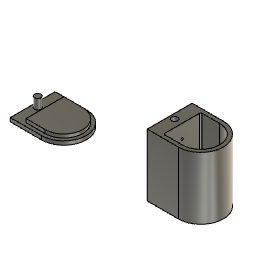
Motor Holder large v1 (Autodesk Fusion 360 design; units mm, degrees)
Autodesk Fusion 360 part; units mm, degrees
sketch "Sketch1" plane through (0, 0, 0) normal (0, 0, 1) x (1, 0, 0)
  line L0 (0, 0) -> (0, 36)
  line L1 (0, 18) -> (18, 18) construction
  circle A0 centre (18, 18) radius 18
  line L2 (0, 36) -> (18, 36)
  line L3 (0, 0) -> (18, 0)
  circle A1 centre (18, 18) radius 1
  circle A2 centre (97.408, 18) radius 1
  line L4 (79.408, 18) -> (97.408, 18) construction
  line L5 (79.408, 36) -> (97.408, 36)
  line L6 (79.408, 0) -> (79.408, 36)
  circle A3 centre (97.408, 18) radius 18
  line L7 (79.408, 0) -> (97.408, 0)
  line L8 (0, 0) -> (-7, 0)
  line L9 (-7, 0) -> (-7, 36)
  line L10 (-7, 36) -> (0, 36)
  line L11 (-117, 0) -> (-117, 36)
  line L12 (-117, 36) -> (-110, 36)
  line L13 (-110, 0) -> (-92, 0)
  line L14 (-110, 0) -> (-117, 0)
  circle A4 centre (-92, 18) radius 18
  line L15 (-110, 18) -> (-92, 18) construction
  line L16 (-110, 0) -> (-110, 36)
  line L17 (-110, 36) -> (-92, 36)
  point P0 (79.408, 0)
  point P1 (-110, 0)
  dimension "d1" = 36
  dimension "d2" = 18
  dimension "d8" = 2
  dimension "d21" = 36
  dimension "d22" = 18
  dimension "d23" = 2
  dimension "d24" = 7
  dimension "d25" = 36
  dimension "d26" = 18
  dimension "d28" = 7
  constraint vertical L0
  constraint coincident L0.start L3.start
  constraint midpoint L0 L1.start
  constraint perpendicular L0 L1
  constraint coincident L1.end A0.centre
  constraint coincident L1.start A0
  constraint coincident A0 L2.end
  constraint tangent A0 L2
  constraint coincident A0 L3.end
  constraint tangent A0 L3
  constraint concentric A0 A1
  constraint vertical L6
  constraint coincident P0 L6.start
  constraint midpoint L4.start L6
  constraint perpendicular L4 L6
  constraint coincident A2.centre L4.end
  constraint coincident L4.start A3
  constraint coincident L5.end A3
  constraint tangent L5 A3
  constraint coincident L7.end A3
  constraint tangent A3 L7
  constraint concentric A2 A3
  constraint perpendicular L0 L8
  constraint perpendicular L8 L9
  constraint vertical L16
  constraint coincident P1 L13.start
  constraint midpoint L15.start L16
  constraint perpendicular L15 L16
  constraint coincident A4.centre L15.end
  constraint coincident L15.start A4
  constraint coincident L17.end A4
  constraint tangent A4 L17
  constraint coincident L13.end A4
  constraint tangent L13 A4
  constraint perpendicular L14 L16
  constraint perpendicular L11 L14
  measures "d1" distance of L0.start L0.end
  measures "d2" distance of L1.start L1.end
  measures "d8" diameter of A1
  measures "d21" distance of P0 L5.start
  measures "d22" distance of A2.centre L4.start
  measures "d23" diameter of A2
  measures "d24" distance of L0.start L8.end
  measures "d25" distance of P1 L12.end
  measures "d26" distance of A4.centre L15.start
  measures "d28" distance of P1 L11.start
extrude "Extrude6" add sketch "Sketch1" along normal blind 3 contours L13 A4 L16 | A4 L16 L17 | A4 makes body 1
extrude "Extrude1" add sketch "Sketch1" along normal blind 50 separate body contours L0 A0 L3 | L0 A0 L2 | A0 | A1 makes body 2
shell "Shell1" thickness 3 removed faces 1 at (19.9503, 20.9653, 50) on bodies 2
sketch "Sketch2" plane through (0, 0, 0) normal (-1, 0, 0) x (0, -1, 0)
  line L0 (-36, 0) -> (0, 0)
  line L1 (0, 0) -> (0, 50)
  line L2 (0, 50) -> (-36, 50)
  line L3 (-36, 50) -> (-36, 0)
  line L4 (-18, 50) -> (-18, 39) construction
  circle A0 centre (-18, 39) radius 1
  dimension "d13" = 11
  dimension "d14" = 2
  constraint midpoint L2 L4.start
  constraint perpendicular L2 L4
  constraint coincident L4.end A0.centre
  measures "d13" distance of L4.start L4.end
  measures "d14" diameter of A0
extrude "Extrude2" add sketch "Sketch2" along normal blind 7 contours L0 L1 L2 L3 | A0 bodies 2
extrude "Extrude3" cut sketch "Sketch1" along normal blind 3 contours A1 bodies 2
extrude "Extrude4" cut sketch "Sketch1" 1 faces at (1, 18, 0) against normal blind 1 contours L0 A0 L3 | L0 A0 L2 | A0 on bodies 2 bodies 2
extrude "Extrude5" cut sketch "Sketch2" along normal blind 14 and the other way blind 7 contours A0 bodies 2
fillet "Fillet1" radius 1 6 edges at (3, 3, 26.5) (3, 33, 26.5) (3, 18, 3) (10.5, 33, 3) (33, 18, 3) (10.5, 3, 3) on bodies 2
extrude "Extrude7" add 1 faces at (-104, 30, 3) along direction (0, 0, 1) blind 2 on bodies 1 bodies 1
shell "Shell2" thickness 2.8 removed faces 1 at (-86.1504, 16.6649, 5) on bodies 1
sketch "Sketch3" plane through (0, 0, 2.8) normal (0, 0, 1) x (-1, 0, 0)
  line L0 (107.2, -2.8) -> (92, -2.8)
  arc A0 (92, -2.8) -> (92, -33.2) centre (92, -18) ccw
  line L1 (92, -33.2) -> (107.2, -33.2)
  line L2 (107.2, -33.2) -> (107.2, -2.8)
extrude "Extrude8" add sketch "Sketch3" along normal blind 3 bodies 1
extrude "Extrude9" cut 1 faces at (-109.0667, 12.9333, 5) along direction (0, 0, -1) blind 2 on bodies 1 bodies 1
extrude "Extrude10" add sketch "Sketch1" along normal blind 3 contours L11 L12 L14 L16 bodies 1
sketch "Sketch4" plane through (0, 0, 50) normal (0, 0, 1) x (-1, 0, 0)
  line L0 (-4, -33) -> (-18, -33)
  arc A0 (-18, -3) -> (-18, -33) centre (-18, -18) ccw
  line L1 (-18, -3) -> (-4, -3)
  arc A1 (-3, -4) -> (-4, -3) centre (-4, -4) ccw
  line L2 (-3, -4) -> (-3, -32)
  arc A2 (-4, -33) -> (-3, -32) centre (-4, -32) ccw
  line L3 (7, 0) -> (-18, 0)
  arc A3 (-18, 0) -> (-18, -36) centre (-18, -18) ccw
  line L4 (-18, -36) -> (7, -36)
  line L5 (7, -36) -> (7, 0)
  line L6 (7, -18) -> (3, -18) construction
  circle A4 centre (3, -18) radius 2.5
  dimension "d40" = 4
  dimension "d41" = 5
  constraint midpoint L5 L6.start
  constraint perpendicular L2 L6
  constraint coincident L6.end A4.centre
  measures "d40" distance of L6.start L6.end
  measures "d41" diameter of A4
extrude "Extrude11" cut sketch "Sketch4" against normal blind 8 contours A4 bodies 2
sketch "Sketch5" plane through (0, 0, 3) normal (0, 0, 1) x (-1, 0, 0)
  line L0 (107.2, -2.8) -> (107.2, -33.2)
  line L1 (107.2, -33.2) -> (92, -33.2)
  arc A0 (92, -2.8) -> (92, -33.2) centre (92, -18) ccw
  line L2 (92, -2.8) -> (107.2, -2.8)
  line L3 (117, 0) -> (92, 0)
  arc A1 (92, 0) -> (92, -36) centre (92, -18) ccw
  line L4 (92, -36) -> (110, -36)
  line L5 (110, -36) -> (117, -36)
  line L6 (117, -36) -> (117, 0)
  line L7 (117, -18) -> (113, -18) construction
  circle A2 centre (113, -18) radius 2.55
  dimension "d44" = 5.1
  constraint midpoint L6 L7.start
  constraint perpendicular L6 L7
  constraint coincident L7.end A2.centre
  measures "d44" diameter of A2
extrude "Extrude12" add sketch "Sketch5" along normal blind 8 contours A2 bodies 1
